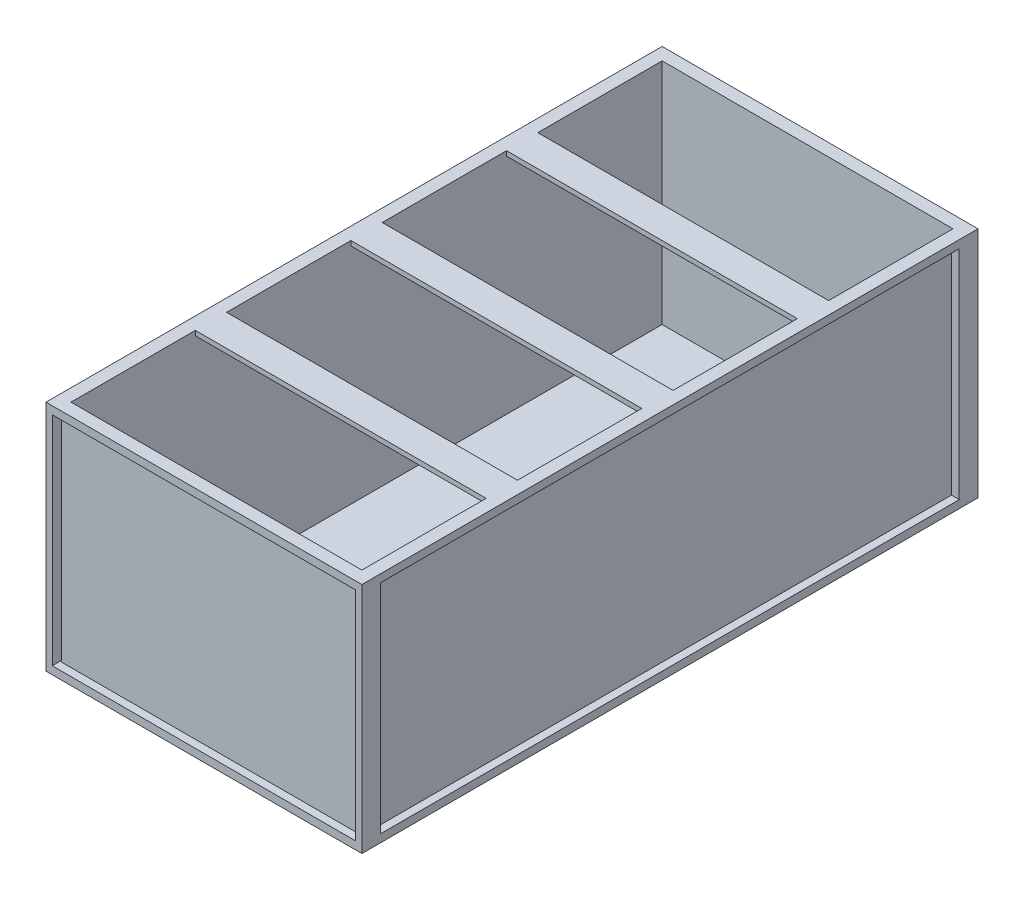
# Autodesk Inventor part: CustomAquariumsTank
Saved by Autodesk Inventor 2022 (Build 260153000, 153)
## iProperties
Created: 2021-06-23
Part Number: CustomAquariumsTank
Material: Generic
Document SubType Name: Modeling
Designer: jamieson-bl
Density: 1 g/cm^3
Appearance: Default
Mass: 215463 g
Surface Area: 220556 cm^2
Volume: 215463 cm^3
Author: jamieson-bl
Autodesk Inventor part; units mm, degrees
ref_plane "YZ Plane" through (0, 0, 0) normal (1, 0, 0) x (0, 1, 0)
ref_plane "XZ Plane" through (0, 0, 0) normal (0, 1, 0) x (-1, 0, 0)
ref_plane "XY Plane" through (0, 0, 0) normal (0, 0, 1) x (1, 0, 0)
sketch "Sketch1" plane through (0, 0, 0) normal (0, 1, 0) x (-1, 0, 0)
  line L0 (-609.6, -1219.2) -> (609.6, -1219.2)
  line L1 (609.6, -1219.2) -> (609.6, 1219.2)
  line L2 (609.6, 1219.2) -> (-609.6, 1219.2)
  line L3 (-609.6, 1219.2) -> (-609.6, -1219.2)
  line L4 (-609.6, -1219.2) -> (609.6, 1219.2) construction
  line L5 (609.6, -1219.2) -> (-609.6, 1219.2) construction
  point P0 (0, 0)
  dimension "d0" = 1219.2
  dimension "d1" = 2438.4
  constraints: 12 end point, 2 midpoint, 2 parallel, 1 horizontal, 1 perpendicular
  measures "d0" distance of L2.end L1.end
  measures "d1" distance of L1.end L0.end
extrude "Extrusion1" add sketch "Sketch1" along normal blind 914.4
sketch "Sketch2" plane through (0, 914.4, 0) normal (0, 1, 0) x (1, 0, 0)
  line L0 (590.55, 1200.15) -> (-590.55, 1200.15)
  line L1 (-590.55, 1200.15) -> (-590.55, -1200.15)
  line L2 (-590.55, -1200.15) -> (590.55, -1200.15)
  line L3 (590.55, -1200.15) -> (590.55, 1200.15)
  line L4 (590.55, 1200.15) -> (-590.55, -1200.15) construction
  line L5 (-590.55, 1200.15) -> (590.55, -1200.15) construction
  point P0 (0, 0)
  dimension "d4" = 1181.1
  dimension "d5" = 2400.3
  constraints: 12 end point, 2 midpoint, 2 parallel, 1 horizontal, 1 perpendicular
  measures "d4" distance of L2.end L1.end
  measures "d5" distance of L1.end L0.end
extrude "Extrusion2" cut sketch "Sketch2" against normal blind 895.35
sketch "Sketch3" plane through (0, 914.4, 0) normal (0, 1, 0) x (1, 0, 0)
  line L0 (641.35, 1250.95) -> (-641.35, 1250.95)
  line L1 (-641.35, 1250.95) -> (-641.35, -1250.95)
  line L2 (-641.35, -1250.95) -> (641.35, -1250.95)
  line L3 (641.35, -1250.95) -> (641.35, 1250.95)
  line L4 (641.35, 1250.95) -> (-641.35, -1250.95) construction
  line L5 (-641.35, 1250.95) -> (641.35, -1250.95) construction
  line L6 (-590.55, -1200.15) -> (-590.55, 1200.15) projected
  line L7 (590.55, 1200.15) -> (-590.55, 1200.15)
  line L8 (-590.55, 1200.15) -> (-590.55, -1200.15)
  line L9 (-590.55, -1200.15) -> (590.55, -1200.15)
  line L10 (590.55, -1200.15) -> (590.55, 1200.15)
  line L11 (590.55, 1200.15) -> (-590.55, -1200.15) construction
  line L12 (-590.55, 1200.15) -> (590.55, -1200.15) construction
  point P0 (0, 0)
  point P1 (-590.55, 1200.15)
  dimension "d8" = 1282.7
  dimension "d9" = 2501.9
  constraints: 24 end point, 4 midpoint, 4 parallel, 2 horizontal, 2 perpendicular
  measures "d8" distance of L2.end L1.end
  measures "d9" distance of L1.end L0.end
extrude "Extrusion3" add sketch "Sketch3" along normal blind 31.75
pattern_linear "Rectangular Pattern1" count 2 spacing 914.4 along (0, -1, 0) of "Extrusion3"
sketch "Sketch4" plane through (-641.35, 31.75, 1250.95) normal (0, 1, 0) x (1, 0, 0)
  line L0 (0, 0) -> (1282.7, 0) projected
  line L1 (1282.7, 0) -> (1282.7, 76.2)
  line L2 (1282.7, 0) -> (1282.7, 2501.9) projected
  line L3 (1282.7, 76.2) -> (1231.9, 76.2)
  line L4 (1231.9, 2451.1) -> (1231.9, 50.8) projected
  line L5 (1231.9, 76.2) -> (1231.9, 50.8)
  line L6 (1231.9, 50.8) -> (1257.3, 50.8)
  line L7 (1231.9, 50.8) -> (50.8, 50.8) projected
  line L8 (1257.3, 50.8) -> (1257.3, 0)
  line L9 (1257.3, 0) -> (1282.7, 0)
  point P0 (641.35, 1250.95)
  point P1 (1257.3, 0)
  dimension "d15" = 76.2
  dimension "d16" = 50.8
  dimension "d17" = 25.4
  dimension "d23" = 25.4
  dimension "d24" = 50.8
  dimension "d25" = 25.4
  constraints: 12 end point, 3 point on line, 2 perpendicular, 1 collinear
  measures "d15" distance of L0.end L1.end
  measures "d16" distance of L1.end L3.end
  measures "d17" distance of L4.end L6.end
  measures "d23" distance of L3.end L4.end
  measures "d24" distance between parallel lines of L0 L7
  measures "d25" distance between parallel lines of L1 L8
extrude "Extrusion4" add sketch "Sketch4" along normal blind 889
mirror "Mirror2" about plane through (0, 0, 0) normal (1, 0, 0) of "Extrusion4"
mirror "Mirror3" about plane through (0, 0, 0) normal (0, 0, 1) of "Extrusion4", "Mirror2"
sketch "Sketch5" plane through (0, 946.15, 0) normal (0, 1, 0) x (1, 0, 0)
  line L0 (-590.55, -1200.15) -> (-590.55, 1200.15) projected
  line L1 (590.55, -695.325) -> (-590.55, -695.325)
  line L2 (-590.55, -695.325) -> (-590.55, -568.325)
  line L3 (-590.55, -568.325) -> (590.55, -568.325)
  line L4 (590.55, -568.325) -> (590.55, -695.325)
  line L5 (590.55, -695.325) -> (-590.55, -568.325) construction
  line L6 (-590.55, -695.325) -> (590.55, -568.325) construction
  line L7 (590.55, 695.325) -> (-590.55, 695.325)
  line L8 (-590.55, 695.325) -> (-590.55, 568.325)
  line L9 (-590.55, 568.325) -> (590.55, 568.325)
  line L10 (590.55, 568.325) -> (590.55, 695.325)
  line L11 (590.55, 695.325) -> (-590.55, 568.325) construction
  line L12 (-590.55, 695.325) -> (590.55, 568.325) construction
  line L13 (590.55, -63.5) -> (-590.55, -63.5)
  line L14 (-590.55, -63.5) -> (-590.55, 63.5)
  line L15 (-590.55, 63.5) -> (590.55, 63.5)
  line L16 (590.55, 63.5) -> (590.55, -63.5)
  line L17 (590.55, -63.5) -> (-590.55, 63.5) construction
  line L18 (-590.55, -63.5) -> (590.55, 63.5) construction
  line L19 (-590.55, 1200.15) -> (590.55, 1200.15) projected
  line L20 (590.55, -1200.15) -> (-590.55, -1200.15) projected
  point P0 (0, 0)
  point P1 (0, -631.825)
  point P2 (0, 631.825)
  point P3 (-590.55, -63.5)
  point P4 (-590.55, 695.325)
  dimension "d26" = 127
  dimension "d27" = 127
  dimension "d28" = 127
  dimension "d31" = 504.825
  dimension "d32" = 504.825
  dimension "d33" = 504.825
  dimension "d34" = 504.825
  constraints: 36 end point, 6 midpoint, 6 parallel, 3 horizontal, 3 perpendicular, 3 point on line
  measures "d26" distance of L1.end L2.end
  measures "d27" distance of L8.end L7.end
  measures "d28" distance of L13.end L14.end
  measures "d31" distance between parallel lines of L7 L19
  measures "d32" distance between parallel lines of L15 L9
  measures "d33" distance between parallel lines of L3 L13
  measures "d34" distance between parallel lines of L20 L1
extrude "Extrusion5" add sketch "Sketch5" against normal blind 19.05
body "Solid1"
